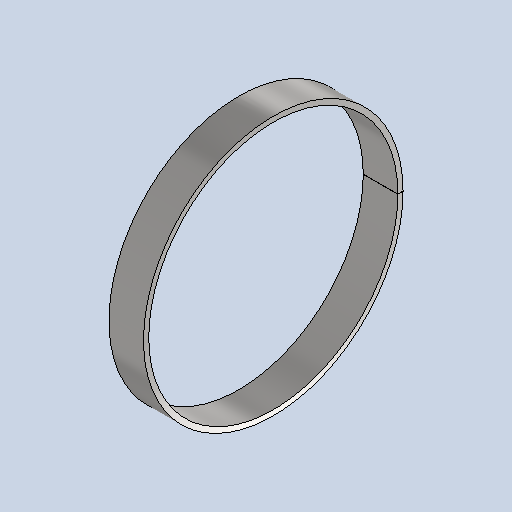
# Autodesk Inventor part: MSC 405 FLANGE COVER RING 500
Saved by Autodesk Inventor 2025 (Build 290162010, 162A)
## iProperties
Created: 2024-06-25
Part Number: MSC 405 FLANGE COVER RING 500
Material: Stainless Steel
Document SubType Name: Sheet Metal
Designer: pokla
Density: 8 g/cm^3
Sheet Metal Rule: AISI304 3mm Die 32
Appearance: Semi-Polished
Flat Pattern Width: 2 cm
Flat Pattern Length: 46.0555 cm
Flat Pattern Area: 92.111 cm^2
Sheet Metal Width: 20,000 mm
Sheet Metal Length: 460,555 mm
Sheet Metal Area: 9211,104 mm^2
Stock Number: МОО 405 усилитель крышки фланца 500 кольцо
Mass: 221.609 g
Surface Area: 213.575 cm^2
Volume: 27.7012 cm^3
Author: pokla
Autodesk Inventor part; units mm, degrees
ref_plane "YZ Plane" through (0, 0, 0) normal (1, 0, 0) x (0, 1, 0)
ref_plane "XZ Plane" through (0, 0, 0) normal (0, 1, 0) x (-1, 0, 0)
ref_plane "XY Plane" through (0, 0, 0) normal (0, 0, 1) x (1, 0, 0)
sketch "Sketch1" plane through (0, 0, 0) normal (0, 0, 1) x (1, 0, 0)
  line L0 (-10, 75) -> (10, 75)
  line L1 (10, 75) -> (10, 72)
  line L2 (10, 72) -> (-10, 72)
  line L3 (-10, 72) -> (-10, 75)
  line L4 (-14, 0) -> (14, 0) projected
  point P0 (0, 0)
  point P1 (0, 75)
  dimension "d2" = 3
  dimension "d3" = 20
  dimension "d4" = 75
  constraints: 8 end point, 2 parallel, 1 horizontal, 1 midpoint, 1 perpendicular, 1 vertical alignment
  measures "d2" distance of L0.end L1.end
  measures "d3" distance of L0.start L0.end
  measures "d4" distance from line of point (0, 0) L0
revolve "Revolution1" add sketch "Sketch1" angle 359.9 about axis through (-10, 0, 0) along (1, 0, 0)
equation "\"BendReliefWidth\" = Thickness"
equation "\"BendReliefDepth\" = 0.5 * Thickness"
equation "\"CornerReliefSize\" = 4 * Thickness"
equation "\"MinimumRemnant\" = 2 * Thickness"
equation "\"TransitionRadius\" = BendRadius"
equation "\"JacobiRadiusSize\" = BendRadius"
equation "\"GapSize\" = Thickness"
equation "\"Thickness\" = 3"
equation "\"BendRadius\" = 5"
body "Solid1"
